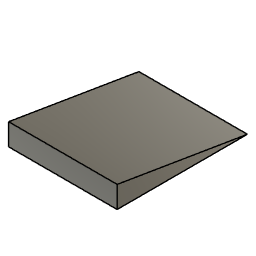
Door Holder (Autodesk Fusion 360 design; units mm, degrees)
Autodesk Fusion 360 part; units mm, degrees
sketch "Sketch1" plane through (0, 0, 0) normal (0, 0, 1) x (1, 0, 0)
  line L0 (25, -30) -> (-25, -30)
  line L1 (-25, -30) -> (-25, 30)
  line L2 (-25, 30) -> (25, 30)
  line L3 (25, 30) -> (25, -30)
  line L4 (25, -30) -> (-25, 30) construction
  line L5 (-25, -30) -> (25, 30) construction
  dimension "d1" = 50
  dimension "d2" = 60
  constraint horizontal L0
  constraint perpendicular L0 L1
  constraint parallel L0 L2
  constraint parallel L1 L3
  constraint coincident L4 origin
  constraint coincident L5 origin
  measures "d1" distance of L1 L3
  measures "d2" distance of L0 L2
extrude "Extrude1" add sketch "Sketch1" along normal blind 10
sketch "Sketch2" plane through (25, 0, 0) normal (1, 0, 0) x (0, 1, 0)
  line L0 (-30, 0) -> (30, 0)
  line L1 (30, 0) -> (30, 10)
  line L2 (30, 10) -> (-30, 10)
  line L3 (-30, 10) -> (-30, 0)
  line L4 (-30, 10) -> (30, 0)
  line L5 (30, 10) -> (-30, 10)
  constraint coincident L2.end L3.start
  constraint coincident L0.end L1.start
  constraint coincident L1.end L2.start
extrude "Extrude2" cut sketch "Sketch2" against normal blind 50 contours L1 L2 L4 L5
